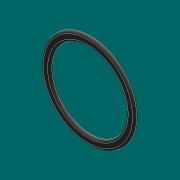
# Autodesk Inventor part: oRing
Saved by Autodesk Inventor 2016 (Build 200138000, 138)
## iProperties
Created: 2016-09-24
Part Number: oRing
Material: Rubber
Document SubType Name: Modeling
Designer: sawaiz
Density: 0.93 g/cm^3
Appearance: Rubber - Black
Author: sawaiz
Autodesk Inventor part; units mm, degrees
ref_plane "YZ Plane" through (0, 0, 0) normal (1, 0, 0) x (0, 1, 0)
ref_plane "XZ Plane" through (0, 0, 0) normal (0, 1, 0) x (-1, 0, 0)
ref_plane "XY Plane" through (0, 0, 0) normal (0, 0, 1) x (1, 0, 0)
sketch "Sketch1" plane through (0, 0, 0) normal (0, 1, 0) x (-1, 0, 0)
  circle A0 centre (0, 0) radius 11.1252
  circle A1 centre (0, 0) radius 13.6652
  dimension "d0" = 22.2504
  dimension "d1" = 2.54
  constraints: 2 centre point, 1 coincident
  measures "d0" diameter of A0
  measures "d1" radial gap between concentric circles of A0 A1
extrude "Extrusion1" add sketch "Sketch1" along normal blind 1.2446
fillet "Fillet1" radius 0.635 4 edges at (13.6652, 1.2446, 0) (11.1252, 1.2446, 0) (13.6652, 0, 0) (11.1252, 0, 0)
equation "\"d0\" = oRingID"
equation "\"d1\" = oRingGrooveWidth"
equation "\"d2\" = oRingGrooveDepth"
equation "\"tubeHeight\" = 50.8"
equation "\"tubeWidth\" = 152.4"
equation "\"tubeLength\" = 304.8"
equation "\"tubeWallThickness\" = 3.175"
equation "\"plateOverhang\" = 6.35"
equation "\"moatWidth\" = 3.175"
equation "\"moatDepth\" = 3.175"
equation "\"tubePlateClearance\" = 0.127"
equation "\"blankCapThickness\" = 9.525"
equation "\"sensorCapThickness\" = 12.7"
equation "\"glassTubeDiameter\" = 12.7"
equation "\"glassTubeClearance\" = 0.19844"
equation "\"longHoleSpacing\" = 30.48"
equation "\"shortHoleSpacing\" = 21.59"
equation "\"sensorHolderDiameter\" = 50.8"
equation "\"sensorHolderThickness\" = 12.7"
equation "\"fiberDiameter\" = 1"
equation "\"fiberClearance\" = 0"
equation "\"oRingID\" = 22.2504"
equation "\"oRingGrooveWidth\" = 2.54"
equation "\"oRingGrooveDepth\" = 1.2446"
equation "\"glassTubeLength\" = 279.4"
equation "\"glassTubeID\" = 7.874"
equation "\"sensorBoardHoleSpacing\" = 19"
body "Solid1"
